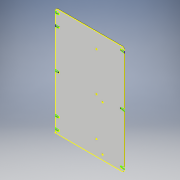
# Autodesk Inventor part: MainBoard
Saved by Autodesk Inventor 2019 (Build 230136000, 136)
## iProperties
Created: 2020-09-12
Part Number: MainBoard
Material: Generic
Document SubType Name: Modeling
Designer: johnh
Density: 1 g/cm^3
Appearance: Default
Author: johnh
Autodesk Inventor part; units mm, degrees
ref_plane "YZ Plane" through (0, 0, 0) normal (1, 0, 0) x (0, 1, 0)
ref_plane "XZ Plane" through (0, 0, 0) normal (0, 1, 0) x (-1, 0, 0)
ref_plane "XY Plane" through (0, 0, 0) normal (0, 0, 1) x (1, 0, 0)
sketch "Sketch1" plane through (0, 0, 0) normal (0, 0, 1) x (1, 0, 0)
  line L0 (0, 0) -> (177.8, 0)
  line L1 (177.8, 0) -> (177.8, 279.4)
  line L2 (177.8, 279.4) -> (0, 279.4)
  line L3 (0, 279.4) -> (0, 0)
  line L4 (8.89, 279.4) -> (168.91, 279.4)
  line L5 (168.91, 0) -> (8.89, 0)
  circle A0 centre (8.89, 139.7) radius 1.6828
  circle A1 centre (8.89, 269.875) radius 1.6828
  circle A2 centre (8.89, 9.525) radius 1.6827
  circle A3 centre (168.91, 9.525) radius 1.6827
  circle A4 centre (168.91, 139.7) radius 1.6827
  circle A5 centre (168.91, 269.875) radius 1.6828
  line L6 (13.843, 279.4) -> (163.957, 279.4)
  line L7 (163.957, 0) -> (13.843, 0)
  circle A6 centre (8.89, 240.03) radius 1.6828
  circle A7 centre (8.89, 39.37) radius 1.6828
  circle A8 centre (105.918, 39.37) radius 1.6827
  circle A9 centre (105.918, 139.7) radius 1.6827
  circle A10 centre (105.918, 240.03) radius 1.6828
  circle A11 centre (121.539, 12.7) radius 1.6827
  circle A12 centre (121.539, 129.54) radius 1.6828
  dimension "d0" = 177.8
  dimension "d1" = 279.4
  dimension "d12" = 3.3655
  dimension "d15" = 3.3655
  dimension "d16" = 3.3655
  dimension "d17" = 3.3655
  dimension "d18" = 3.3655
  dimension "d19" = 3.3655
  dimension "d27" = 3.3655
  dimension "d28" = 3.3655
  dimension "d31" = 3.3655
  dimension "d32" = 3.3655
  dimension "d33" = 3.3655
  dimension "d42" = 3.3655
  dimension "d43" = 3.3655
  dimension "d50" = 8.89
  dimension "d51" = 105.918
  dimension "d52" = 121.539
  dimension "d53" = 168.91
  dimension "d54" = 9.525
  dimension "d55" = 39.37
  dimension "d56" = 12.7
  dimension "d57" = 139.7
  dimension "d58" = 129.54
  dimension "d59" = 240.03
  dimension "d60" = 269.875
  constraints: 16 end point, 13 centre point, 4 parallel, 4 point on line, 3 horizontal, 2 vertical alignment, 1 perpendicular
  measures "d0" distance of L2.end L1.end
  measures "d1" distance of L1.end L0.end
  measures "d12" diameter of A0
  measures "d15" diameter of A1
  measures "d16" diameter of A2
  measures "d17" diameter of A3
  measures "d18" diameter of A4
  measures "d19" diameter of A5
  measures "d27" diameter of A6
  measures "d28" diameter of A7
  measures "d31" diameter of A8
  measures "d32" diameter of A9
  measures "d33" diameter of A10
  measures "d42" diameter of A11
  measures "d43" diameter of A12
  measures "d50" distance from line of L3 A1.centre
  measures "d51" distance from line of A10.centre L3
  measures "d52" distance from line of L3 A12.centre
  measures "d53" distance from line of L3 A3.centre
  measures "d54" distance of L5.start A3.centre
  measures "d55" distance from line of L0 A8.centre
  measures "d56" distance from line of L0 A11.centre
  measures "d57" distance from line of L0 A9.centre
  measures "d58" distance from line of L0 A12.centre
  measures "d59" distance from line of L0 A10.centre
  measures "d60" distance from line of L0 A5.centre
extrude "Extrusion1" add sketch "Sketch1" along normal blind 1.27
fillet "Fillet1" radius 6.35 4 edges at (0, 279.4, 0.635) (177.8, 279.4, 0.635) (0, 0, 0.635) (177.8, 0, 0.635)
sketch "Sketch2" plane through (0, 0, 1.27) normal (0, 0, 1) x (1, 0, 0)
  arc A0 (171.45, 0) -> (177.8, 6.35) centre (171.45, 6.35) ccw projected
  line L0 (177.8, 6.35) -> (177.8, 273.05) projected
  arc A1 (177.8, 273.05) -> (171.45, 279.4) centre (171.45, 273.05) ccw projected
  line L1 (171.45, 279.4) -> (6.35, 279.4) projected
  arc A2 (6.35, 279.4) -> (0, 273.05) centre (6.35, 273.05) ccw projected
  line L2 (0, 273.05) -> (0, 6.35) projected
  arc A3 (0, 6.35) -> (6.35, 0) centre (6.35, 6.35) ccw projected
  line L3 (6.35, 0) -> (171.45, 0) projected
  circle A4 centre (121.539, 129.54) radius 1.6828 projected
  circle A5 centre (121.539, 12.7) radius 1.6827 projected
  circle A6 centre (105.918, 240.03) radius 1.6828 projected
  circle A7 centre (105.918, 139.7) radius 1.6827 projected
  circle A8 centre (105.918, 39.37) radius 1.6827 projected
  circle A9 centre (8.89, 39.37) radius 1.6828 projected
  circle A10 centre (8.89, 240.03) radius 1.6828 projected
  circle A11 centre (168.91, 269.875) radius 1.6828 projected
  circle A12 centre (168.91, 139.7) radius 1.6827 projected
  circle A13 centre (168.91, 9.525) radius 1.6827 projected
  circle A14 centre (8.89, 9.525) radius 1.6827 projected
  circle A15 centre (8.89, 269.875) radius 1.6828 projected
  circle A16 centre (8.89, 139.7) radius 1.6828 projected
  line L4 (8.89, 141.3827) -> (0, 142.4743)
  line L5 (8.89, 138.0173) -> (0, 136.9257)
  line L6 (0, 142.4743) -> (0, 136.9257)
  arc A17 (8.89, 141.3827) -> (8.89, 138.0173) centre (8.89, 139.7) ccw
  line L7 (8.89, 141.3827) -> (0, 142.4743)
  line L8 (8.89, 138.0173) -> (0, 136.9257)
  line L9 (0, 142.4743) -> (0, 136.9257)
  arc A18 (8.89, 141.3827) -> (8.89, 138.0173) centre (8.89, 139.7) ccw
  line L10 (8.89, 241.7127) -> (0, 242.8043)
  line L11 (8.89, 238.3472) -> (0, 237.2557)
  line L12 (0, 242.8043) -> (0, 237.2557)
  arc A19 (8.89, 241.7127) -> (8.89, 238.3472) centre (8.89, 240.03) ccw
  line L13 (8.89, 271.5577) -> (0, 272.6493)
  line L14 (8.89, 268.1922) -> (0, 267.1007)
  line L15 (0, 272.6493) -> (0, 267.1007)
  arc A20 (8.89, 271.5577) -> (8.89, 268.1922) centre (8.89, 269.875) ccw
  line L16 (8.89, 41.0527) -> (0, 42.1443)
  line L17 (8.89, 37.6872) -> (0, 36.5957)
  line L18 (0, 42.1443) -> (0, 36.5957)
  arc A21 (8.89, 41.0527) -> (8.89, 37.6872) centre (8.89, 39.37) ccw
  line L19 (8.89, 11.2077) -> (0, 12.2993)
  line L20 (8.89, 7.8422) -> (0, 6.7507)
  line L21 (0, 12.2993) -> (0, 6.7507)
  arc A22 (8.89, 11.2077) -> (8.89, 7.8422) centre (8.89, 9.525) ccw
  line L22 (168.91, 138.0173) -> (177.8, 136.9257)
  line L23 (168.91, 141.3827) -> (177.8, 142.4743)
  line L24 (177.8, 136.9257) -> (177.8, 142.4743)
  arc A23 (168.91, 138.0173) -> (168.91, 141.3827) centre (168.91, 139.7) ccw
  line L25 (168.91, 138.0173) -> (177.8, 136.9257)
  line L26 (168.91, 141.3827) -> (177.8, 142.4743)
  line L27 (177.8, 136.9257) -> (177.8, 142.4743)
  arc A24 (168.91, 138.0173) -> (168.91, 141.3827) centre (168.91, 139.7) ccw
  line L28 (168.91, 268.1923) -> (177.8, 267.1007)
  line L29 (168.91, 271.5577) -> (177.8, 272.6493)
  line L30 (177.8, 267.1007) -> (177.8, 272.6493)
  arc A25 (168.91, 268.1923) -> (168.91, 271.5577) centre (168.91, 269.875) ccw
  line L31 (168.91, 7.8423) -> (177.8, 6.7507)
  line L32 (168.91, 11.2078) -> (177.8, 12.2993)
  line L33 (177.8, 6.7507) -> (177.8, 12.2993)
  arc A26 (168.91, 7.8423) -> (168.91, 11.2078) centre (168.91, 9.525) ccw
  point P0 (0, 0)
  constraints: 60 end point, 24 point on circle, 10 centre point, 6 vertical, 4 point on line, 2 concentric, 1 collinear
extrude "Extrusion2" cut sketch "Sketch2" against normal blind 1.27 contours L31 A13 L32 L0 | L22 A12 L23 L0 | L2 L4 A16 L5 | L2 L13 A15 L14
sketch "Sketch3" plane through (0, 0, 1.27) normal (0, 0, 1) x (1, 0, 0)
  circle A0 centre (8.89, 9.525) radius 1.6827 projected
  circle A1 centre (168.91, 269.875) radius 1.6828 projected
  circle A2 centre (8.89, 240.03) radius 1.6828 projected
  circle A3 centre (8.89, 39.37) radius 1.6828 projected
  circle A4 centre (105.918, 39.37) radius 1.6827 projected
  circle A5 centre (105.918, 139.7) radius 1.6827 projected
  circle A6 centre (105.918, 240.03) radius 1.6828 projected
  circle A7 centre (121.539, 12.7) radius 1.6827 projected
  circle A8 centre (121.539, 129.54) radius 1.6828 projected
  line L0 (8.89, 268.1922) -> (0, 267.1007) projected
  line L1 (0, 267.1007) -> (0, 142.4743) projected
  line L2 (0, 142.4743) -> (8.89, 141.3827) projected
  arc A9 (8.89, 138.0173) -> (8.89, 141.3827) centre (8.89, 139.7) ccw projected
  line L3 (8.89, 138.0173) -> (0, 136.9257) projected
  line L4 (0, 136.9257) -> (0, 6.35) projected
  arc A10 (0, 6.35) -> (6.35, 0) centre (6.35, 6.35) ccw projected
  line L5 (6.35, 0) -> (171.45, 0) projected
  arc A11 (171.45, 0) -> (177.8, 6.35) centre (171.45, 6.35) ccw projected
  line L6 (177.8, 6.35) -> (177.8, 6.7507) projected
  line L7 (177.8, 6.7507) -> (168.91, 7.8423) projected
  arc A12 (168.91, 11.2078) -> (168.91, 7.8423) centre (168.91, 9.525) ccw projected
  line L8 (168.91, 11.2078) -> (177.8, 12.2993) projected
  line L9 (177.8, 12.2993) -> (177.8, 136.9257) projected
  line L10 (177.8, 136.9257) -> (168.91, 138.0173) projected
  arc A13 (168.91, 141.3827) -> (168.91, 138.0173) centre (168.91, 139.7) ccw projected
  line L11 (168.91, 141.3827) -> (177.8, 142.4743) projected
  line L12 (177.8, 142.4743) -> (177.8, 273.05) projected
  arc A14 (177.8, 273.05) -> (171.45, 279.4) centre (171.45, 273.05) ccw projected
  line L13 (171.45, 279.4) -> (6.35, 279.4) projected
  arc A15 (6.35, 279.4) -> (0, 273.05) centre (6.35, 273.05) ccw projected
  line L14 (0, 273.05) -> (0, 272.6493) projected
  line L15 (0, 272.6493) -> (8.89, 271.5577) projected
  arc A16 (8.89, 268.1922) -> (8.89, 271.5577) centre (8.89, 269.875) ccw projected
  line L16 (8.89, 11.2077) -> (0, 12.2993)
  line L17 (0, 12.2993) -> (0, 6.7507)
  line L18 (0, 6.7507) -> (8.89, 7.8422)
  arc A17 (8.89, 11.2077) -> (8.89, 7.8422) centre (8.89, 9.525) ccw
  point P0 (0, 0)
  constraints: 6 end point, 4 point on circle, 2 point on line, 1 centre point, 1 concentric
extrude "Extrusion3" cut sketch "Sketch3" against normal blind 1.27 contours A0 L18 L4 L16
sketch "Sketch4" plane through (0, 0, 1.27) normal (0, 0, 1) x (1, 0, 0)
  circle A0 centre (121.539, 129.54) radius 1.6828 projected
  circle A1 centre (121.539, 12.7) radius 1.6827 projected
  circle A2 centre (105.918, 240.03) radius 1.6828 projected
  circle A3 centre (105.918, 139.7) radius 1.6827 projected
  circle A4 centre (105.918, 39.37) radius 1.6827 projected
  circle A5 centre (8.89, 39.37) radius 1.6828 projected
  circle A6 centre (8.89, 240.03) radius 1.6828 projected
  circle A7 centre (168.91, 269.875) radius 1.6828 projected
  line L0 (8.89, 7.8422) -> (0, 6.7507) projected
  line L1 (0, 6.7507) -> (0, 6.35) projected
  arc A8 (0, 6.35) -> (6.35, 0) centre (6.35, 6.35) ccw projected
  line L2 (6.35, 0) -> (171.45, 0) projected
  arc A9 (171.45, 0) -> (177.8, 6.35) centre (171.45, 6.35) ccw projected
  line L3 (177.8, 6.35) -> (177.8, 6.7507) projected
  line L4 (177.8, 6.7507) -> (168.91, 7.8423) projected
  arc A10 (168.91, 11.2078) -> (168.91, 7.8423) centre (168.91, 9.525) ccw projected
  line L5 (168.91, 11.2078) -> (177.8, 12.2993) projected
  line L6 (177.8, 12.2993) -> (177.8, 136.9257) projected
  line L7 (177.8, 136.9257) -> (168.91, 138.0173) projected
  arc A11 (168.91, 141.3827) -> (168.91, 138.0173) centre (168.91, 139.7) ccw projected
  line L8 (168.91, 141.3827) -> (177.8, 142.4743) projected
  line L9 (177.8, 142.4743) -> (177.8, 273.05) projected
  arc A12 (177.8, 273.05) -> (171.45, 279.4) centre (171.45, 273.05) ccw projected
  line L10 (171.45, 279.4) -> (6.35, 279.4) projected
  arc A13 (6.35, 279.4) -> (0, 273.05) centre (6.35, 273.05) ccw projected
  line L11 (0, 273.05) -> (0, 272.6493) projected
  line L12 (0, 272.6493) -> (8.89, 271.5577) projected
  arc A14 (8.89, 268.1922) -> (8.89, 271.5577) centre (8.89, 269.875) ccw projected
  line L13 (8.89, 268.1922) -> (0, 267.1007) projected
  line L14 (0, 267.1007) -> (0, 142.4743) projected
  line L15 (0, 142.4743) -> (8.89, 141.3827) projected
  arc A15 (8.89, 138.0173) -> (8.89, 141.3827) centre (8.89, 139.7) ccw projected
  line L16 (8.89, 138.0173) -> (0, 136.9257) projected
  line L17 (0, 136.9257) -> (0, 12.2993) projected
  line L18 (0, 12.2993) -> (8.89, 11.2077) projected
  arc A16 (8.89, 7.8422) -> (8.89, 11.2077) centre (8.89, 9.525) ccw projected
  line L19 (8.89, 41.0527) -> (0, 42.1443)
  line L20 (8.89, 37.6872) -> (0, 36.5957)
  line L21 (0, 42.1443) -> (0, 36.5957)
  arc A17 (8.89, 41.0527) -> (8.89, 37.6872) centre (8.89, 39.37) ccw
  line L22 (8.89, 241.7127) -> (0, 242.8043)
  line L23 (8.89, 238.3472) -> (0, 237.2557)
  line L24 (0, 237.2557) -> (0, 242.8043)
  arc A18 (8.89, 241.7127) -> (8.89, 238.3472) centre (8.89, 240.03) ccw
  line L25 (168.91, 271.5577) -> (177.8, 272.6493)
  line L26 (168.91, 268.1923) -> (177.8, 267.1007)
  line L27 (177.8, 267.1007) -> (177.8, 272.6493)
  arc A19 (168.91, 268.1923) -> (168.91, 271.5577) centre (168.91, 269.875) ccw
  point P0 (0, 0)
  constraints: 18 end point, 13 point on circle, 6 point on line, 5 concentric, 3 centre point, 2 collinear, 1 vertical
extrude "Extrusion4" cut sketch "Sketch2" against normal blind 1.27 contours L2 L16 A9 L17 | L28 A11 L29 L0 | L2 L10 A10 L11
body "Solid1"
